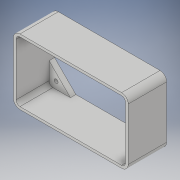
# Autodesk Inventor part: THAD Back
Saved by Autodesk Inventor 2018 (Build 220112000, 112)
## iProperties
Created: 2018-11-08
Part Number: THAD Back
Material: Generic
Document SubType Name: Modeling
Designer: joshj
Density: 1 g/cm^3
Appearance: Default
Author: joshj
Autodesk Inventor part; units mm, degrees
ref_plane "YZ Plane" through (0, 0, 0) normal (1, 0, 0) x (0, 1, 0)
ref_plane "XZ Plane" through (0, 0, 0) normal (0, 1, 0) x (-1, 0, 0)
ref_plane "XY Plane" through (0, 0, 0) normal (0, 0, 1) x (1, 0, 0)
sketch "Sketch1" plane through (0, 0, 0) normal (0, 0, 1) x (1, 0, 0)
  line L0 (0, 0) -> (209.2, 0)
  line L1 (209.2, 0) -> (209.2, 119.3)
  line L2 (209.2, 119.3) -> (0, 119.3)
  line L3 (0, 119.3) -> (0, 0)
  dimension "d0" = 209.2
  dimension "d1" = 119.3
  constraints: 8 end point, 2 perpendicular, 1 horizontal, 1 vertical
  measures "d0" distance of L0.start L0.end
  measures "d1" distance of L0.end L1.end
extrude "Extrusion1" add sketch "Sketch1" along normal blind 10
fillet "Fillet1" radius 12 4 edges at (209.2, 119.3, 5) (209.2, 0, 5) (0, 119.3, 5) (0, 0, 5)
sketch "Sketch3" plane through (0, 0, 10) normal (0, 0, 1) x (1, 0, 0)
  circle A0 centre (18, 101.602) radius 3.5
  line L0 (0, 107.3) -> (0, 12) projected
  line L1 (197.2, 119.3) -> (12, 119.3) projected
  line L2 (197.2, 119.3) -> (12, 119.3) construction
  line L3 (104.6, 119.3) -> (104.6, 0) construction
  line L4 (12, 0) -> (197.2, 0) construction
  circle A1 centre (191.2, 101.602) radius 3.5
  line L5 (0, 59.65) -> (209.2, 59.65) construction
  line L6 (209.2, 12) -> (209.2, 107.3) construction
  circle A2 centre (18, 17.698) radius 3.5
  circle A3 centre (191.2, 17.698) radius 3.5
  point P0 (0, 0)
  dimension "d16" = 7
  dimension "d17" = 18
  dimension "d18" = 17.698
  constraints: 4 centre point, 4 end point, 4 midpoint, 3 symmetric about line, 3 other
  measures "d16" diameter of A0
  measures "d17" distance from line of L0 A0.centre
  measures "d18" distance from line of L1 A0.centre
extrude "Extrusion3" cut sketch "Sketch3" against normal through all
sketch "Sketch4" plane through (0, 0, 10) normal (0, 0, 1) x (1, 0, 0)
  circle A0 centre (18, 101.602) radius 3.5 construction
  line L0 (18, 101.602) -> (18, 119.3) construction
  line L1 (12, 119.3) -> (24, 119.3)
  arc A1 (12, 119.3) -> (0, 107.3) centre (12, 107.3) ccw projected
  line L2 (0, 107.3) -> (0, 95.3)
  line L3 (197.2, 119.3) -> (12, 119.3) construction
  line L4 (104.6, 119.3) -> (104.6, 0) construction
  line L5 (12, 0) -> (197.2, 0) construction
  line L6 (0, 107.3) -> (0, 12) construction
  line L7 (0, 59.65) -> (209.2, 59.65) construction
  line L8 (209.2, 12) -> (209.2, 107.3) construction
  line L9 (191.2, 101.602) -> (191.2, 119.3) construction
  line L10 (197.2, 119.3) -> (185.2, 119.3)
  arc A2 (209.2, 107.3) -> (197.2, 119.3) centre (197.2, 107.3) ccw
  line L11 (209.2, 107.3) -> (209.2, 95.3)
  line L12 (12, 0) -> (24, 0)
  arc A3 (0, 12) -> (12, 0) centre (12, 12) ccw
  line L13 (0, 12) -> (0, 24)
  line L14 (197.2, 0) -> (12, 0) construction
  line L15 (197.2, 0) -> (185.2, 0)
  line L16 (209.2, 12) -> (209.2, 24)
  arc A4 (197.2, 0) -> (209.2, 12) centre (197.2, 12) ccw
  line L17 (24, 0) -> (185.2, 0)
  line L18 (0, 95.3) -> (0, 24)
  line L19 (209.2, 93.9155) -> (209.2, 24)
  line L20 (209.2, 12) -> (209.2, 107.3) projected
  line L21 (197.2, 119.3) -> (12, 119.3) projected
  line L22 (24, 119.3) -> (197.2, 119.3)
  point P0 (0, 0)
  point P1 (104.6, 107.3)
  point P2 (12, 59.65)
  point P3 (18, 17.698)
  point P4 (191.2, 17.698)
  dimension "d21" = 12
  dimension "d22" = 12
  constraints: 34 end point, 13 symmetric about line, 6 point on circle, 4 collinear, 4 midpoint, 3 centre point, 3 point on line, 1 vertical, 3 other
  measures "d21" distance of L1.start L1.end
  measures "d22" distance of L2.start L2.end
extrude "Extrusion4" cut sketch "Sketch4" against normal blind 10 keep common part
sketch "Sketch5" plane through (0, 0, 10) normal (0, 0, 1) x (1, 0, 0)
  line L0 (43.891, 114.602) -> (165.309, 114.602)
  line L1 (43.891, 4.698) -> (165.309, 4.698)
  line L2 (12, 0) -> (197.2, 0) projected
  line L3 (104.6, 107.3) -> (104.6, 0) construction
  line L4 (43.891, 114.602) -> (5, 75.7075)
  line L5 (5, 43.5925) -> (5, 75.7075)
  line L6 (5, 43.5925) -> (43.891, 4.698)
  line L7 (165.309, 114.602) -> (204.2, 75.7075)
  line L8 (204.2, 43.5925) -> (204.2, 75.7075)
  line L9 (204.2, 43.5925) -> (165.309, 4.698)
  line L10 (0, 107.3) -> (0, 12) projected
  line L11 (0, 59.65) -> (209.2, 59.65) construction
  line L12 (209.2, 12) -> (209.2, 107.3) construction
  line L13 (197.2, 119.3) -> (12, 119.3) construction
  point P0 (0, 0)
  point P1 (104.6, 114.602)
  point P2 (5, 59.65)
  dimension "d25" = 4.698
  dimension "d27" = 121.418
  dimension "d37" = 5
  dimension "d38" = 32.115
  dimension "d39" = 4.698
  constraints: 20 end point, 5 midpoint, 2 point on line, 2 symmetric about line, 1 horizontal, 1 parallel, 1 vertical
  measures "d25" distance between parallel lines of L2 L1
  measures "d27" distance of L0.start L0.end
  measures "d37" distance between parallel lines of L10 L5
  measures "d38" distance of L5.start L4.end
  measures "d39" distance between parallel lines of L13 L0
extrude "Extrusion5" cut sketch "Sketch5" against normal through all
sketch "Sketch8" plane through (0, 0, 10) normal (0, 0, 1) x (1, 0, 0)
  line L0 (197.2, 119.3) -> (12, 119.3) projected
  line L1 (12, 119.3) -> (197.2, 119.3)
  line L2 (209.2, 12) -> (209.2, 107.3) projected
  line L3 (209.2, 107.3) -> (209.2, 12)
  line L4 (12, 0) -> (197.2, 0) projected
  line L5 (197.2, 0) -> (12, 0)
  line L6 (0, 107.3) -> (0, 12) projected
  line L7 (0, 107.3) -> (0, 12)
  arc A0 (12, 119.3) -> (0, 107.3) centre (12, 107.3) ccw projected
  arc A1 (209.2, 107.3) -> (197.2, 119.3) centre (197.2, 107.3) ccw projected
  arc A2 (197.2, 0) -> (209.2, 12) centre (197.2, 12) ccw projected
  arc A3 (0, 12) -> (12, 0) centre (12, 12) ccw projected
  line L8 (5, 75.7075) -> (5, 12)
  line L9 (5, 75.7075) -> (5, 107.3)
  line L10 (165.309, 4.698) -> (43.891, 4.698) projected
  line L11 (43.891, 4.698) -> (12, 4.698)
  line L12 (165.309, 4.698) -> (197.2, 4.698)
  line L13 (204.2, 43.5925) -> (204.2, 75.7075) projected
  line L14 (204.2, 75.7075) -> (204.2, 12)
  line L15 (204.2, 75.7075) -> (204.2, 107.3)
  line L16 (43.891, 114.602) -> (197.2, 114.602)
  line L17 (43.891, 114.602) -> (165.309, 114.602) projected
  line L18 (43.891, 114.602) -> (12, 114.602)
  arc A4 (5, 12) -> (12, 4.698) centre (12.3085, 12) ccw
  arc A5 (197.2, 4.698) -> (204.2, 12) centre (196.8915, 12) ccw
  arc A6 (204.2, 107.3) -> (197.2, 114.602) centre (197.2, 107.5958) ccw
  arc A7 (12, 114.602) -> (5, 107.3) centre (12, 107.5958) ccw
  point P0 (0, 0)
  constraints: 24 end point, 8 point on circle, 6 collinear, 4 centre point, 4 tangent, 3 horizontal, 3 vertical
extrude "Extrusion7" add sketch "Sketch8" along normal blind 60
body "Solid1"
